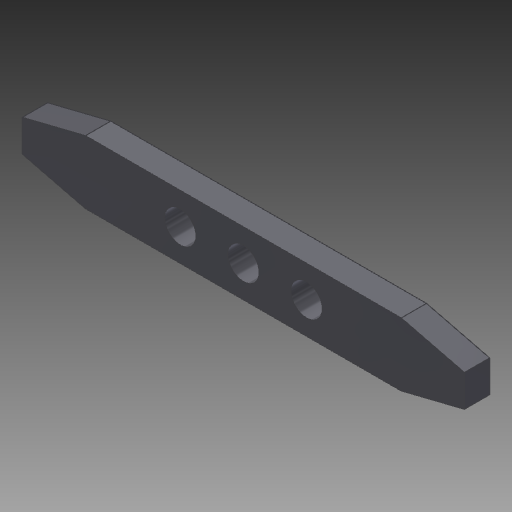
# Autodesk Inventor part: J001375
Saved by Autodesk Inventor 2018.2 (Build 222227000, 227)
## iProperties
Created: 2012-11-09
Material: TITANIUM, 6AL-4V, ANNEALED
Vendor: HHMI: JFRC - ID&F
Document SubType Name: Modeling
Designer: OSBORNEJ
Density: 4.43 g/cm^3
Part Number: J001375
Project: P-091902
Description: KS STYLE HEADPOST WITH THREE EPOXY HOLES MOUSE HEAD POST
Mass: 0.278213 g
Surface Area: 1.70994 cm^2
Volume: 0.062802 cm^3
Appearance: Metal-Steel (Polished)
RuleStatus: InUse
AfterDocSave0: file://Part Number Cleaner
LAB/DEPT: COMMON
REQUESTING SCIENTIST: COMMON
SURFACE ROUGHNESS: 63RA
DESIGN DEPARTMENT: HHMI: JRC - ID&F
SPECIAL FINISH: NONE
ALTERED ITEM PART NUMBER: N/A
ALTERED ITEM VENDOR: N/A
ALTERED ITEM DESCRIPTION: N/A
Revision Number: -
Autodesk Inventor part; units mm, degrees
ref_plane "YZ Plane" through (0, 0, 0) normal (1, 0, 0) x (0, 1, 0)
ref_plane "XZ Plane" through (0, 0, 0) normal (0, 1, 0) x (-1, 0, 0)
ref_plane "XY Plane" through (0, 0, 0) normal (0, 0, 1) x (1, 0, 0)
sketch "Sketch1" plane through (0, 0, 0) normal (0, 0, 1) x (1, 0, 0)
  line L0 (-11.1125, 1.5875) -> (11.1125, 1.5875)
  line L1 (11.1125, 1.5875) -> (11.1125, -1.5875)
  line L2 (11.1125, -1.5875) -> (-11.1125, -1.5875)
  line L3 (-11.1125, -1.5875) -> (-11.1125, 1.5875)
  line L4 (-7.9375, 1.5875) -> (-11.1125, 0.8001)
  line L5 (-7.9375, -1.5875) -> (-11.1125, -0.8001)
  line L6 (7.9375, -1.5875) -> (11.1125, -0.8001)
  line L7 (11.1125, 0.8001) -> (7.9375, 1.5875)
  point P0 (0, 0)
  point P1 (-3.175, 0)
  point P2 (0, 0)
  point P3 (3.175, 0)
  dimension "d0" = 3.175
  dimension "d1" = 22.225
  dimension "d2" = 11.1125
  dimension "d3" = 1.5875
  dimension "d4" = 1.6002
  dimension "d5" = 1.6002
  dimension "d6" = 0.7874
  dimension "d7" = 0.7874
  dimension "d8" = 3.175
  dimension "d9" = 3.175
  dimension "d10" = 3.175
  dimension "d11" = 3.175
  dimension "d12" = 3.175
  dimension "d13" = 3.175
  dimension "d14" = 0
  dimension "d15" = 1.5875
  constraints: 16 end point, 8 point on line, 2 parallel, 1 coincident, 1 horizontal, 1 perpendicular
  measures "d0" distance of L0.end L1.end
  measures "d1" distance of L0.start L0.end
  measures "d2" distance from line of point (0, 0) L1
  measures "d3" distance from line of point (0, 0) L0
  measures "d4" distance of L5.end L4.end
  measures "d5" distance of L7.start L6.end
  measures "d6" distance of L5.end L2.end
  measures "d7" distance of L6.end L1.end
  measures "d8" distance from line of L6.start L1
  measures "d9" distance from line of L7.end L1
  measures "d10" horizontal distance of L4.start L4.end
  measures "d11" horizontal distance of L5.end L5.start
  measures "d12" distance of point (3.175, 0) point (0, 0)
  measures "d13" distance of point (0, 0) point (-3.175, 0)
  measures "d14" vertical distance of point (-3.175, 0) point (0, 0)
  measures "d15" distance from line of L2 point (3.175, 0)
extrude "Extrusion1" add sketch "Sketch1" along normal blind 1.27 contours L0 L7 L1 L6 L2 L5 L3 L4
hole "Hole1" at (-3.175, 0, 0) at (0, 0, 0) at (3.175, 0, 0) direction (0, 0, 1) diameter 1.6002 end through all
equation "\"d2\" = 0.5 * d1"
equation "\"d3\" = 0.5 * d0"
body "Solid1"
